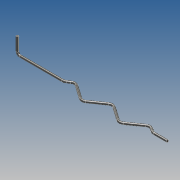
# Autodesk Inventor part: Barra expulsora 1
Saved by Autodesk Inventor 2016 (Build 200138000, 138)
## iProperties
Created: 2016-05-25
Part Number: Barra expulsora 1
Material: Stainless Steel
Document SubType Name: Modeling
Designer: Familia
Density: 8 g/cm^3
Appearance: Chrome - Polished
Mass: 7.53417 g
Surface Area: 15.1665 cm^2
Volume: 0.941772 cm^3
Author: Familia
Autodesk Inventor part; units mm, degrees
ref_plane "YZ Plane" through (0, 0, 0) normal (1, 0, 0) x (0, 1, 0)
ref_plane "XZ Plane" through (0, 0, 0) normal (0, 1, 0) x (-1, 0, 0)
sketch "Sketch1" plane through (0, 0, 0) normal (0, 0, 1) x (1, 0, 0)
  line L0 (0, 0) -> (48.4239, 0)
  line L1 (51.2912, 0.9038) -> (54.2755, 2.9929)
  line L2 (60.0102, 2.9929) -> (74.2755, -6.9929)
  line L3 (80.0102, -6.9929) -> (94.2755, 2.9929)
  line L4 (100.0102, 2.9929) -> (114.2755, -6.9929)
  line L5 (120.0102, -6.9929) -> (134.2755, 2.9929)
  line L6 (140.0102, 2.9929) -> (142.9945, 0.9038)
  line L7 (157.1429, -9) -> (160, -7) construction
  line L8 (145.8618, 0) -> (160, 0)
  arc A0 (48.4239, 0) -> (51.2912, 0.9038) centre (48.4239, 5) ccw
  arc A1 (60.0102, 2.9929) -> (54.2755, 2.9929) centre (57.1429, -1.1033) ccw
  arc A2 (74.2755, -6.9929) -> (80.0102, -6.9929) centre (77.1429, -2.8967) ccw
  arc A3 (100.0102, 2.9929) -> (94.2755, 2.9929) centre (97.1429, -1.1033) ccw
  arc A4 (114.2755, -6.9929) -> (120.0102, -6.9929) centre (117.1429, -2.8967) ccw
  arc A5 (140.0102, 2.9929) -> (134.2755, 2.9929) centre (137.1429, -1.1033) ccw
  arc A6 (142.9945, 0.9038) -> (145.8618, 0) centre (145.8618, 5) ccw
  point P0 (50, 0)
  point P1 (57.1429, 5)
  point P2 (77.1429, -9)
  point P3 (97.1429, 5)
  point P4 (117.1429, -9)
  point P5 (137.1429, 5)
  point P6 (144.2857, 0)
  dimension "d0" = 160
  dimension "d1" = 50
  dimension "d2" = 20
  dimension "d3" = 20
  dimension "d4" = 20
  dimension "d5" = 20
  dimension "d6" = 20
  dimension "d7" = 14
  dimension "d8" = 5
  dimension "d9" = 15.7143
  dimension "d14" = 5
  constraints: 18 end point, 14 point on circle, 14 point on line, 14 tangent, 7 centre point, 6 equal radius, 4 horizontal alignment, 2 horizontal, 2 parallel, 1 collinear, 1 vertical alignment
  measures "d0" horizontal distance of L7.end L0.start
  measures "d1" distance of L0.start point (50, 0)
  measures "d2" horizontal distance of point (77.143, -9) point (57.143, 5)
  measures "d3" horizontal distance of point (97.143, 5) point (77.143, -9)
  measures "d4" horizontal distance of point (117.143, -9) point (97.143, 5)
  measures "d5" horizontal distance of point (137.143, 5) point (117.143, -9)
  measures "d6" horizontal distance of L7.start point (137.143, 5)
  measures "d7" vertical distance of point (77.143, -9) point (57.143, 5)
  measures "d8" vertical distance of point (57.143, 5) point (50, 0)
  measures "d9" distance of point (144.286, 0) L8.end
  measures "d14" radius of A0
ref_plane "Work Plane1" through (0, 0, 17) normal (0, 0, 1) x (1, 0, 0)
sketch "Sketch2" plane through (0, 0, 17) normal (0, 0, 1) x (1, 0, 0)
  circle A0 centre (0, 0) radius 1.25
  dimension "d11" = 2.5
  constraints: 1 centre point, 1 coincident
  measures "d11" diameter of A0
sketch3d "3D Sketch1"
  line L0 (0, 0, 17) -> (0, 0, 3)
  arc A0 (0, 0, 3) -> (3, 0, 0) centre (3, 0, 3) ccw
  line L1 (3, 0, 0) -> (48.4239, 0, 0)
  arc A1 (48.4239, 0, 0) -> (51.2912, 0.9038, 0) centre (48.4239, 5, 0) ccw
  line L2 (51.2912, 0.9038, 0) -> (54.2755, 2.9929, 0)
  arc A2 (54.2755, 2.9929, 0) -> (60.0102, 2.9929, 0) centre (57.1429, -1.1033, 0) ccw
  line L3 (60.0102, 2.9929, 0) -> (74.2755, -6.9929, 0)
  arc A3 (74.2755, -6.9929, 0) -> (80.0102, -6.9929, 0) centre (77.1429, -2.8967, 0) ccw
  line L4 (80.0102, -6.9929, 0) -> (94.2755, 2.9929, 0)
  arc A4 (94.2755, 2.9929, 0) -> (100.0102, 2.9929, 0) centre (97.1429, -1.1033, 0) ccw
  line L5 (100.0102, 2.9929, 0) -> (114.2755, -6.9929, 0)
  arc A5 (114.2755, -6.9929, 0) -> (120.0102, -6.9929, 0) centre (117.1429, -2.8967, 0) ccw
  line L6 (120.0102, -6.9929, 0) -> (134.2755, 2.9929, 0)
  arc A6 (134.2755, 2.9929, 0) -> (140.0102, 2.9929, 0) centre (137.1429, -1.1033, 0) ccw
  line L7 (140.0102, 2.9929, 0) -> (142.9945, 0.9038, 0)
  arc A7 (142.9945, 0.9038, 0) -> (145.8618, 0, 0) centre (145.8618, 5, 0) ccw
  line L8 (145.8618, 0, 0) -> (160, 0, 0)
  dimension "d15" = 17
  dimension "d16" = 90
  dimension "d17" = 3
  constraints: 2 vertical
sweep "Sweep2" add profiles "Sketch2" path "3D Sketch1"
body "Solid2"
